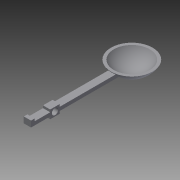
# Autodesk Inventor part: 000205
Saved by Autodesk Inventor 2015 (Build 190159000, 159)
## iProperties
Created: 2015-05-27
Part Number: 000205
Material: Generic
Document SubType Name: Modeling
Designer: Wesley
Density: 1 g/cm^3
Appearance: Default
Author: Wesley
Autodesk Inventor part; units mm, degrees
ref_plane "YZ Plane" through (0, 0, 0) normal (1, 0, 0) x (0, 1, 0)
ref_plane "XZ Plane" through (0, 0, 0) normal (0, 1, 0) x (-1, 0, 0)
sketch "Sketch2" plane through (0, 0, 0) normal (0, 0, 1) x (1, 0, 0)
  arc A0 (0, -12.7) -> (10.9985, -6.35) centre (0, 0) ccw
  arc A1 (0, -11.43) -> (9.5038, -6.35) centre (0, 0) ccw
  line L0 (0, -11.43) -> (0, -12.7)
  line L1 (10.9985, -6.35) -> (9.5038, -6.35)
  dimension "d4" = 25.4
  dimension "d5" = 22.86
  dimension "d9" = 6.35
  dimension "d10" = 10.9985
  constraints: 4 end point, 4 point on circle, 2 centre point, 2 coincident, 1 horizontal, 1 vertical
  measures "d4" diameter of A0
  measures "d5" diameter of A1
  measures "d9" distance from line of L0.end L1
  measures "d10" distance from line of L0 L1.start
revolve "Revolution1" add sketch "Sketch2" angle 360 about axis through (0, -11.43, 0) along (0, -1, 0)
ref_plane "Work Plane1" through (0, 0, 10.795) normal (0, 0, 1) x (1, 0, 0)
sketch "Sketch3" plane through (0, 0, 10.795) normal (0, 0, 1) x (1, 0, 0)
  line L0 (-1.905, -6.985) -> (1.905, -6.985)
  line L1 (1.905, -6.985) -> (1.905, -8.89)
  line L2 (1.905, -8.89) -> (-1.905, -8.89)
  line L3 (-1.905, -8.89) -> (-1.905, -6.985)
  line L4 (-10.9985, -6.35) -> (10.9985, -6.35) projected
  point P0 (0, 0)
  dimension "d12" = 1.905
  dimension "d13" = 1.905
  dimension "d14" = 1.905
  dimension "d15" = 0.635
  constraints: 8 end point, 2 parallel, 1 horizontal, 1 perpendicular
  measures "d12" distance from line of point (0, 0) L3
  measures "d13" distance from line of point (0, 0) L1
  measures "d14" distance between parallel lines of L2 L0
  measures "d15" distance between parallel lines of L4 L0
extrude "Extrusion1" add sketch "Sketch3" along normal blind 44.45
sketch "Sketch4" plane through (0, 0, 10.795) normal (0, 0, -1) x (-1, 0, 0)
  line L0 (1.905, -6.985) -> (-1.905, -6.985) projected
  line L1 (-1.905, -6.985) -> (-1.905, -8.89) projected
  line L2 (-1.905, -8.89) -> (1.905, -8.89) projected
  line L3 (1.905, -8.89) -> (1.905, -6.985) projected
  point P0 (0, 0)
extrude "Extrusion2" add sketch "Sketch4" along normal blind 1.016
sketch "Sketch5" plane through (0, 0, 9.779) normal (0, 0, -1) x (-1, 0, 0)
  line L0 (-1.905, -8.89) -> (1.905, -8.89)
  line L1 (1.905, -8.89) -> (1.905, -7.876)
  line L2 (1.905, -7.876) -> (-1.905, -7.876)
  line L3 (-1.905, -7.876) -> (-1.905, -8.89)
  point P0 (0, 0)
  constraints: 8 end point, 2 parallel, 1 horizontal, 1 perpendicular
extrude "Extrusion3" add sketch "Sketch5" along normal blind 1.016
sketch "Sketch6" plane through (1.905, -8.89, 55.245) normal (1, 0, 0) x (0, 0, -1)
  line L0 (0, 1.905) -> (44.8109, 1.905) projected
  line L1 (0, 0) -> (0, 1.905) projected
  point P0 (55.245, 8.89)
  point P1 (12.7, 0.9525)
  dimension "d24" = 0.9525
  dimension "d25" = 12.7
  measures "d24" distance from line of point (12.7, 0.953) L0
  measures "d25" distance from line of L1 point (12.7, 0.953)
sketch "Sketch7" plane through (0, -6.985, 0) normal (0, 1, 0) x (1, 0, 0)
  line L0 (1.905, -55.245) -> (1.905, -8.8673) projected
  line L1 (-1.905, -10.4341) -> (-1.905, -55.245) projected
  line L2 (1.905, -45.085) -> (-1.905, -45.085)
  line L3 (-1.905, -45.085) -> (-1.905, -40.005)
  line L4 (-1.905, -40.005) -> (1.905, -40.005)
  line L5 (1.905, -40.005) -> (1.905, -45.085)
  line L6 (-9.5339, -42.545) -> (17.5873, -42.545) construction
  line L7 (1.905, -55.245) -> (-1.905, -55.245) construction
  point P0 (0, 0)
  dimension "d26" = 12.7
  dimension "d27" = 2.54
  dimension "d28" = 2.54
  constraints: 10 end point, 2 horizontal, 2 parallel, 2 point on line, 1 perpendicular
  measures "d26" distance between parallel lines of L7 L6
  measures "d27" distance between parallel lines of L2 L6
  measures "d28" distance between parallel lines of L6 L4
extrude "Extrusion4" add sketch "Sketch7" along normal blind 1.27 and the other way blind 3.175
hole "Hole1" at (1.905, -7.9375, 42.545) direction (-1, 0, 0) diameter 3.302 depth 25.4 tip angle 118
sketch "Sketch8" plane through (-1.905, -6.985, 55.245) normal (0, 1, 0) x (1, 0, 0)
  line L0 (3.81, 0) -> (3.81, 10.16) projected
  line L1 (0, 0) -> (3.81, 0)
  line L2 (3.81, 0) -> (3.81, 1.905)
  line L3 (3.81, 1.905) -> (0, 1.905)
  line L4 (0, 1.905) -> (0, 0)
  point P0 (1.905, 55.245)
  dimension "d40" = 1.905
  constraints: 8 end point, 2 parallel, 1 horizontal, 1 perpendicular, 1 point on line
  measures "d40" distance of L2.end L1.end
extrude "Extrusion5" add sketch "Sketch8" along normal blind 1.27
body "Solid1"
